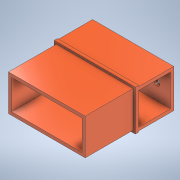
# Autodesk Inventor part: Tapa 51mm
Saved by Autodesk Inventor 2022.6 (Build 266554000, 554)
## iProperties
Created: 2024-09-03
Part Number: Tapa 51mm
Material: Genérico
Document SubType Name: Modeling
Designer: G207
Density: 1 g/cm^3
Appearance: Valor por defecto
Author: G207
Autodesk Inventor part; units mm, degrees
ref_plane "YZ Plane" through (0, 0, 0) normal (1, 0, 0) x (0, 1, 0)
ref_plane "XZ Plane" through (0, 0, 0) normal (0, 1, 0) x (-1, 0, 0)
ref_plane "XY Plane" through (0, 0, 0) normal (0, 0, 1) x (1, 0, 0)
sketch "Boceto1" plane through (0, 0, 0) normal (0, 0, 1) x (1, 0, 0)
  line L0 (0, 0) -> (50.8, 0)
  line L1 (50.8, 0) -> (50.8, 25.4)
  line L2 (50.8, 25.4) -> (0, 25.4)
  line L3 (0, 25.4) -> (0, 0)
  dimension "d0" = 50.8
  dimension "d1" = 25.4
  constraints: 8 end point, 2 parallel, 1 horizontal, 1 perpendicular
  measures "d0" distance of L2.end L1.end
  measures "d1" distance of L1.end L0.end
extrude "Extrusión1" add sketch "Boceto1" along normal blind 2
sketch "Boceto2" plane through (0, 0, 2) normal (0, 0, 1) x (1, 0, 0)
  line L0 (1.4, 1.4) -> (49.4, 1.4)
  line L1 (49.4, 1.4) -> (49.4, 24)
  line L2 (49.4, 24) -> (1.4, 24)
  line L3 (1.4, 24) -> (1.4, 1.4)
  line L4 (0, 25.4) -> (0, 0) projected
  line L5 (0, 0) -> (50.8, 0) projected
  line L6 (50.8, 25.4) -> (0, 25.4) projected
  line L7 (50.8, 0) -> (50.8, 25.4) projected
  line L8 (3.4, 3.4) -> (47.4, 3.4)
  line L9 (47.4, 3.4) -> (47.4, 22)
  line L10 (47.4, 22) -> (3.4, 22)
  line L11 (3.4, 22) -> (3.4, 3.4)
  dimension "d4" = 1.4
  dimension "d5" = 1.4
  dimension "d6" = 1.4
  dimension "d7" = 1.4
  dimension "d8" = 2
  dimension "d9" = 2
  dimension "d10" = 2
  dimension "d11" = 2
  constraints: 16 end point, 4 parallel, 2 horizontal, 2 perpendicular
  measures "d4" distance between parallel lines of L4 L3
  measures "d5" distance between parallel lines of L0 L5
  measures "d6" distance between parallel lines of L6 L2
  measures "d7" distance between parallel lines of L7 L1
  measures "d8" distance between parallel lines of L2 L10
  measures "d9" distance between parallel lines of L8 L0
  measures "d10" distance between parallel lines of L9 L1
  measures "d11" distance between parallel lines of L11 L3
extrude "Extrusión2" add sketch "Boceto2" along normal blind 30 contours L3 L2 L1 L0
sketch "Boceto3" plane through (50.8, 0, 0) normal (1, 0, 0) x (0, 0, -1)
  line L0 (0, 0) -> (0, 25.4) projected
  line L1 (0, 0.7) -> (22, 0.7)
  line L2 (22, 0.7) -> (22, 24.7)
  line L3 (22, 24.7) -> (0, 24.7)
  line L4 (0, 24.7) -> (0, 0.7)
  line L5 (0, 25.4) -> (-2, 25.4) projected
  line L6 (0, 0) -> (-2, 0) projected
  line L7 (0, 2.7) -> (20, 2.7)
  line L8 (20, 2.7) -> (20, 22.7)
  line L9 (20, 22.7) -> (0, 22.7)
  line L10 (0, 22.7) -> (0, 2.7)
  point P0 (-1, 25.4)
  point P1 (0, 24.7)
  point P2 (0, 22.7)
  point P3 (0, 2.7)
  point P4 (0, 0.7)
  dimension "d16" = 24
  dimension "d17" = 25.4
  dimension "d18" = 0.7
  dimension "d19" = 0.7
  dimension "d20" = 22
  dimension "d21" = 0
  dimension "d22" = 2
  dimension "d23" = 2
  dimension "d24" = 2
  dimension "d25" = 20
  dimension "d26" = 20
  constraints: 16 end point, 4 parallel, 2 horizontal, 2 perpendicular, 1 midpoint, 1 point on line
  measures "d16" distance of L1.end L2.end
  measures "d17" distance of L0.start L0.end
  measures "d18" distance from line of L3 point (-1, 25.4)
  measures "d19" distance between parallel lines of L6 L1
  measures "d20" distance of L2.end L3.end
  measures "d21" distance between parallel lines of L4 L0
  measures "d22" distance between parallel lines of L9 L3
  measures "d23" distance between parallel lines of L1 L7
  measures "d24" distance between parallel lines of L2 L8
  measures "d25" distance of L8.end L9.end
  measures "d26" distance of L7.end L8.end
extrude "Extrusión3" add sketch "Boceto3" against normal up to surface (50.8 mm away) contours L0 L7 L8 L9 L3 L2 L1
sketch "Boceto4" plane through (50.8, 0.7, -22) normal (0, 0, -1) x (-1, 0, 0)
  circle A0 centre (8.4, 12) radius 1.75
  circle A1 centre (25.4, 12) radius 1.75
  circle A2 centre (42.4, 12) radius 1.75
  line L0 (50.8, 0) -> (50.8, 24) projected
  line L1 (0, 0) -> (0, 24) projected
  line L2 (0, 0) -> (50.8, 0) projected
  line L3 (0, 24) -> (50.8, 24) projected
  point P0 (50.8, -0.7)
  dimension "d29" = 3.5
  dimension "d30" = 3.5
  dimension "d31" = 3.5
  dimension "d32" = 17
  dimension "d33" = 17
  dimension "d34" = 50.8
  dimension "d39" = 24
  dimension "d40" = 12
  dimension "d41" = 12
  dimension "d42" = 12
  dimension "d43" = 12
  dimension "d44" = 12
  dimension "d45" = 25.4
  dimension "d46" = 8.4
  constraints: 3 centre point
  measures "d29" diameter of A0
  measures "d30" diameter of A1
  measures "d31" diameter of A2
  measures "d32" distance of A1.centre A0.centre
  measures "d33" distance of A2.centre A1.centre
  measures "d34" distance between parallel lines of L0 L1
  measures "d39" distance between parallel lines of L2 L3
  measures "d40" distance from line of A2.centre L3
  measures "d41" distance from line of A1.centre L3
  measures "d42" distance from line of A1.centre L2
  measures "d43" distance from line of L2 A2.centre
  measures "d44" distance from line of L3 A0.centre
  measures "d45" distance from line of A1.centre L1
  measures "d46" distance from line of L0 A2.centre
extrude "Extrusión4" cut sketch "Boceto4" against normal up to surface (2 mm away) contours A0 | A1 | A2
